Autodesk Inventor part; units mm, degrees
(part 2 of 2)
extrude "Cut10" cut sketch "Sketch17" against normal blind 1.5875 contours A302 L31 | L31 A302 L213 A303 L214 | A300 L31 | L31 A300 L211 A301 L212 | A298 L209 A299 L32 E1 L31 | L31 E1 L32 A299 L210 A298 | L234 A322 L233 L33 | L33 L233 L26 L234 | L26 L233 A323 L234 | L232 A320 L231 L33 | L33 L231 L26 L232 | L26 L231 A321 L232 | L247 A337 L248 L37 | L37 L248 A336 L247 | A332 L243 A333 L43 | L43 A333 L244 A332 | A330 L241 A331 L45 | L45 A331 L242 A330 | A201 L112 A200 L51 | L51 A200 L111 A201 | A181 L92 A180 L51 | L51 A180 L91 A181 | A223 L53 | L53 A223 L134 A222 L133 | A225 L53 | L53 A225 L136 A224 L135 | A162 L73 A163 L74 L54 | L54 A162 | A164 L75 A165 L76 L54 | L54 A164 | A207 L118 A206 L52 | L52 A206 L117 A207 | A187 L98 A186 L52 | L52 A186 L97 A187 | A155 L66 A154 L65 | A173 L84 A172 L83 | A175 L86 A174 L85 | A183 L94 A182 L93 | A185 L96 A184 L95 | A193 L104 A192 L103 | A195 L106 A194 L105 | A203 L114 A202 L113 | A205 L116 A204 L115 | A213 L124 A212 L123 | A215 L126 A214 L125 | A233 L144 A232 L143 | A243 L154 A242 L153 | A245 L156 A244 L155 | A263 L174 A262 L173 | A265 L176 A264 L175 | A283 L194 A282 L193 | A285 L196 A284 L195 | A295 L206 A294 L205 | A309 L220 A308 L219 | A315 L226 A314 L225 | A329 L240 A328 L239 | A335 L246 A334 L245 | A339 L250 A338 L249 | A341 L252 A340 L251 | A343 L254 A342 L253 | A345 L256 A344 L255 | A347 L258 A346 L257 | A349 L260 A348 L259
sketch "Sketch19" plane through (0, 0, 1.5875) normal (0, 0, 1) x (1, 0, 0)
  arc A0 (-129.1273, 301.498) -> (-129.1273, 261.3025) centre (-129.1273, 281.4002) ccw projected
  line L0 (-129.1273, 301.498) -> (-112.1728, 301.498) projected
  arc A1 (-112.1728, 261.3025) -> (-112.1728, 301.498) centre (-112.1728, 281.4002) ccw projected
  line L1 (-112.1728, 261.3025) -> (-129.1273, 261.3025) projected
  arc A2 (-192.6273, 301.498) -> (-192.6273, 261.3025) centre (-192.6273, 281.4002) ccw projected
  line L2 (-192.6273, 301.498) -> (-175.6728, 301.498) projected
  arc A3 (-175.6728, 261.3025) -> (-175.6728, 301.498) centre (-175.6728, 281.4002) ccw projected
  line L3 (-175.6728, 261.3025) -> (-192.6273, 261.3025) projected
  arc A4 (-192.6273, 394.589) -> (-192.6273, 354.3935) centre (-192.6273, 374.4912) ccw projected
  line L4 (-192.6273, 394.589) -> (-175.6728, 394.589) projected
  arc A5 (-175.6728, 354.3935) -> (-175.6728, 394.589) centre (-175.6728, 374.4912) ccw projected
  line L5 (-175.6728, 354.3935) -> (-192.6273, 354.3935) projected
  arc A6 (-65.6273, 208.407) -> (-65.6273, 168.2115) centre (-65.6273, 188.3092) ccw projected
  line L6 (-65.6273, 208.407) -> (-48.6728, 208.407) projected
  arc A7 (-48.6728, 168.2115) -> (-48.6728, 208.407) centre (-48.6727, 188.3092) ccw projected
  line L7 (-48.6728, 168.2115) -> (-65.6273, 168.2115) projected
  arc A8 (-65.6273, 301.498) -> (-65.6273, 261.3025) centre (-65.6273, 281.4002) ccw projected
  line L8 (-65.6273, 301.498) -> (-48.6728, 301.498) projected
  arc A9 (-48.6728, 261.3025) -> (-48.6728, 301.498) centre (-48.6727, 281.4002) ccw projected
  line L9 (-48.6728, 261.3025) -> (-65.6273, 261.3025) projected
  arc A10 (-65.6273, 394.589) -> (-65.6273, 354.3935) centre (-65.6273, 374.4913) ccw projected
  line L10 (-65.6273, 394.589) -> (-48.6728, 394.589) projected
  arc A11 (-48.6728, 354.3935) -> (-48.6728, 394.589) centre (-48.6728, 374.4913) ccw projected
  line L11 (-48.6728, 354.3935) -> (-65.6273, 354.3935) projected
  arc A12 (-65.6273, 487.68) -> (-65.6273, 447.4845) centre (-65.6273, 467.5823) ccw projected
  line L12 (-65.6273, 487.68) -> (-48.6728, 487.68) projected
  arc A13 (-48.6728, 447.4845) -> (-48.6728, 487.68) centre (-48.6728, 467.5823) ccw projected
  line L13 (-48.6728, 447.4845) -> (-65.6273, 447.4845) projected
  arc A14 (-129.1273, 115.316) -> (-129.1273, 75.1205) centre (-129.1273, 95.2182) ccw projected
  line L14 (-129.1273, 115.316) -> (-112.1728, 115.316) projected
  arc A15 (-112.1728, 75.1205) -> (-112.1728, 115.316) centre (-112.1728, 95.2182) ccw projected
  line L15 (-112.1728, 75.1205) -> (-129.1273, 75.1205) projected
  arc A16 (-129.1273, 487.68) -> (-129.1273, 447.4845) centre (-129.1273, 467.5822) ccw projected
  line L16 (-129.1273, 487.68) -> (-112.1728, 487.68) projected
  arc A17 (-112.1728, 447.4845) -> (-112.1728, 487.68) centre (-112.1728, 467.5822) ccw projected
  line L17 (-112.1728, 447.4845) -> (-129.1273, 447.4845) projected
  arc A18 (-192.6273, 487.68) -> (-192.6273, 447.4845) centre (-192.6273, 467.5822) ccw projected
  line L18 (-192.6273, 487.68) -> (-175.6728, 487.68) projected
  arc A19 (-175.6728, 447.4845) -> (-175.6728, 487.68) centre (-175.6728, 467.5822) ccw projected
  line L19 (-175.6728, 447.4845) -> (-192.6273, 447.4845) projected
  arc A20 (-256.1273, 301.498) -> (-256.1273, 261.3025) centre (-256.1273, 281.4002) ccw projected
  line L20 (-256.1273, 301.498) -> (-239.1728, 301.498) projected
  arc A21 (-239.1728, 261.3025) -> (-239.1728, 301.498) centre (-239.1728, 281.4002) ccw projected
  line L21 (-239.1728, 261.3025) -> (-256.1273, 261.3025) projected
  arc A22 (-319.6273, 301.498) -> (-319.6273, 261.3025) centre (-319.6273, 281.4002) ccw projected
  line L22 (-319.6273, 301.498) -> (-302.6728, 301.498) projected
  arc A23 (-302.6728, 261.3025) -> (-302.6728, 301.498) centre (-302.6728, 281.4002) ccw projected
  line L23 (-302.6728, 261.3025) -> (-319.6273, 261.3025) projected
  arc A24 (-383.1273, 301.498) -> (-383.1273, 261.3025) centre (-383.1273, 281.4002) ccw projected
  line L24 (-383.1273, 301.498) -> (-366.1728, 301.498) projected
  arc A25 (-366.1728, 261.3025) -> (-366.1728, 301.498) centre (-366.1728, 281.4002) ccw projected
  line L25 (-366.1728, 261.3025) -> (-383.1273, 261.3025) projected
  arc A26 (-446.6273, 254.9525) -> (-446.6273, 214.757) centre (-446.6273, 234.8547) ccw projected
  line L26 (-446.6273, 254.9525) -> (-429.6728, 254.9525) projected
  arc A27 (-429.6728, 214.757) -> (-429.6728, 254.9525) centre (-429.6728, 234.8547) ccw projected
  line L27 (-429.6728, 214.757) -> (-446.6273, 214.757) projected
  arc A28 (-446.6273, 487.68) -> (-446.6273, 447.4845) centre (-446.6273, 467.5822) ccw projected
  line L28 (-446.6273, 487.68) -> (-429.6728, 487.68) projected
  arc A29 (-429.6728, 447.4845) -> (-429.6728, 487.68) centre (-429.6728, 467.5822) ccw projected
  line L29 (-429.6728, 447.4845) -> (-446.6273, 447.4845) projected
  arc A30 (-510.1273, 208.407) -> (-510.1273, 168.2115) centre (-510.1273, 188.3092) ccw projected
  line L30 (-510.1273, 208.407) -> (-493.1728, 208.407) projected
  arc A31 (-493.1728, 168.2115) -> (-493.1728, 208.407) centre (-493.1727, 188.3092) ccw projected
  line L31 (-493.1728, 168.2115) -> (-510.1273, 168.2115) projected
  arc A32 (-510.1273, 301.498) -> (-510.1273, 261.3025) centre (-510.1273, 281.4002) ccw projected
  line L32 (-510.1273, 301.498) -> (-493.1728, 301.498) projected
  arc A33 (-493.1728, 261.3025) -> (-493.1728, 301.498) centre (-493.1728, 281.4002) ccw projected
  line L33 (-493.1728, 261.3025) -> (-510.1273, 261.3025) projected
  arc A34 (-510.1273, 487.68) -> (-510.1273, 447.4845) centre (-510.1273, 467.5822) ccw projected
  line L34 (-510.1273, 487.68) -> (-493.1728, 487.68) projected
  arc A35 (-493.1728, 447.4845) -> (-493.1728, 487.68) centre (-493.1728, 467.5822) ccw projected
  line L35 (-493.1728, 447.4845) -> (-510.1273, 447.4845) projected
  arc A36 (-573.6273, 208.407) -> (-573.6273, 168.2115) centre (-573.6273, 188.3092) ccw projected
  line L36 (-573.6273, 208.407) -> (-556.6728, 208.407) projected
  arc A37 (-556.6728, 168.2115) -> (-556.6728, 208.407) centre (-556.6727, 188.3092) ccw projected
  line L37 (-556.6728, 168.2115) -> (-573.6273, 168.2115) projected
  arc A38 (-573.6273, 301.498) -> (-573.6273, 261.3025) centre (-573.6273, 281.4002) ccw projected
  line L38 (-573.6273, 301.498) -> (-556.6728, 301.498) projected
  arc A39 (-556.6728, 261.3025) -> (-556.6728, 301.498) centre (-556.6728, 281.4002) ccw projected
  line L39 (-556.6728, 261.3025) -> (-573.6273, 261.3025) projected
  arc A40 (-573.6273, 487.68) -> (-573.6273, 447.4845) centre (-573.6273, 467.5822) ccw projected
  line L40 (-573.6273, 487.68) -> (-556.6728, 487.68) projected
  arc A41 (-556.6728, 447.4845) -> (-556.6728, 487.68) centre (-556.6728, 467.5822) ccw projected
  line L41 (-556.6728, 447.4845) -> (-573.6273, 447.4845) projected
  arc A42 (-637.1273, 254.9525) -> (-637.1273, 214.757) centre (-637.1273, 234.8547) ccw projected
  line L42 (-637.1273, 254.9525) -> (-620.1728, 254.9525) projected
  arc A43 (-620.1728, 214.757) -> (-620.1728, 254.9525) centre (-620.1727, 234.8547) ccw projected
  line L43 (-620.1728, 214.757) -> (-637.1273, 214.757) projected
  arc A44 (-637.1273, 487.68) -> (-637.1273, 447.4845) centre (-637.1273, 467.5822) ccw projected
  line L44 (-637.1273, 487.68) -> (-620.1728, 487.68) projected
  arc A45 (-620.1728, 447.4845) -> (-620.1728, 487.68) centre (-620.1728, 467.5822) ccw projected
  line L45 (-620.1728, 447.4845) -> (-637.1273, 447.4845) projected
  arc A46 (-637.1273, 301.498) -> (-637.1273, 261.3025) centre (-637.1273, 281.4002) ccw projected
  line L46 (-637.1273, 301.498) -> (-620.1728, 301.498) projected
  arc A47 (-620.1728, 261.3025) -> (-620.1728, 301.498) centre (-620.1727, 281.4002) ccw projected
  line L47 (-620.1728, 261.3025) -> (-637.1273, 261.3025) projected
  arc A48 (-637.1272, 68.7705) -> (-637.1272, 28.575) centre (-637.1272, 48.6727) ccw projected
  line L48 (-637.1272, 68.7705) -> (-620.1728, 68.7705) projected
  arc A49 (-620.1728, 28.575) -> (-620.1728, 68.7705) centre (-620.1727, 48.6727) ccw projected
  line L49 (-620.1728, 28.575) -> (-637.1272, 28.575) projected
  arc A50 (-573.6273, 348.0435) -> (-573.6273, 307.848) centre (-573.6273, 327.9457) ccw projected
  line L50 (-573.6273, 348.0435) -> (-556.6728, 348.0435) projected
  arc A51 (-556.6728, 307.848) -> (-556.6728, 348.0435) centre (-556.6728, 327.9457) ccw projected
  line L51 (-556.6728, 307.848) -> (-573.6273, 307.848) projected
  arc A52 (-573.6273, 254.9525) -> (-573.6273, 214.757) centre (-573.6273, 234.8547) ccw projected
  line L52 (-573.6273, 254.9525) -> (-556.6728, 254.9525) projected
  arc A53 (-556.6728, 214.757) -> (-556.6728, 254.9525) centre (-556.6727, 234.8547) ccw projected
  line L53 (-556.6728, 214.757) -> (-573.6273, 214.757) projected
  arc A54 (-573.6273, 68.7705) -> (-573.6273, 28.575) centre (-573.6273, 48.6727) ccw projected
  line L54 (-573.6273, 68.7705) -> (-556.6728, 68.7705) projected
  arc A55 (-556.6728, 28.575) -> (-556.6728, 68.7705) centre (-556.6727, 48.6727) ccw projected
  line L55 (-556.6728, 28.575) -> (-573.6273, 28.575) projected
  arc A56 (-510.1273, 348.0435) -> (-510.1273, 307.848) centre (-510.1273, 327.9457) ccw projected
  line L56 (-510.1273, 348.0435) -> (-493.1728, 348.0435) projected
  arc A57 (-493.1728, 307.848) -> (-493.1728, 348.0435) centre (-493.1728, 327.9457) ccw projected
  line L57 (-493.1728, 307.848) -> (-510.1273, 307.848) projected
  arc A58 (-510.1273, 254.9525) -> (-510.1273, 214.757) centre (-510.1273, 234.8547) ccw projected
  line L58 (-510.1273, 254.9525) -> (-493.1728, 254.9525) projected
  arc A59 (-493.1728, 214.757) -> (-493.1728, 254.9525) centre (-493.1727, 234.8547) ccw projected
  line L59 (-493.1728, 214.757) -> (-510.1273, 214.757) projected
  arc A60 (-510.1272, 68.7705) -> (-510.1272, 28.575) centre (-510.1272, 48.6727) ccw projected
  line L60 (-510.1272, 68.7705) -> (-493.1728, 68.7705) projected
  arc A61 (-493.1728, 28.575) -> (-493.1728, 68.7705) centre (-493.1727, 48.6727) ccw projected
  line L61 (-493.1728, 28.575) -> (-510.1272, 28.575) projected
  arc A62 (-446.6273, 301.498) -> (-446.6273, 261.3025) centre (-446.6273, 281.4002) ccw projected
  line L62 (-446.6273, 301.498) -> (-429.6728, 301.498) projected
  arc A63 (-429.6728, 261.3025) -> (-429.6728, 301.498) centre (-429.6728, 281.4002) ccw projected
  line L63 (-429.6728, 261.3025) -> (-446.6273, 261.3025) projected
  arc A64 (-446.6272, 68.7705) -> (-446.6272, 28.575) centre (-446.6272, 48.6727) ccw projected
  line L64 (-446.6272, 68.7705) -> (-429.6728, 68.7705) projected
  arc A65 (-429.6728, 28.575) -> (-429.6728, 68.7705) centre (-429.6728, 48.6727) ccw projected
  line L65 (-429.6728, 28.575) -> (-446.6272, 28.575) projected
  arc A66 (-383.1273, 254.9525) -> (-383.1273, 214.757) centre (-383.1273, 234.8547) ccw projected
  line L66 (-383.1273, 254.9525) -> (-366.1728, 254.9525) projected
  arc A67 (-366.1728, 214.757) -> (-366.1728, 254.9525) centre (-366.1728, 234.8547) ccw projected
  line L67 (-366.1728, 214.757) -> (-383.1273, 214.757) projected
  arc A68 (-319.6273, 254.9525) -> (-319.6273, 214.757) centre (-319.6273, 234.8547) ccw projected
  line L68 (-319.6273, 254.9525) -> (-302.6728, 254.9525) projected
  arc A69 (-302.6728, 214.757) -> (-302.6728, 254.9525) centre (-302.6727, 234.8547) ccw projected
  line L69 (-302.6728, 214.757) -> (-319.6273, 214.757) projected
  arc A70 (-256.1273, 254.9525) -> (-256.1273, 214.757) centre (-256.1273, 234.8547) ccw projected
  line L70 (-256.1273, 254.9525) -> (-239.1728, 254.9525) projected
  arc A71 (-239.1728, 214.757) -> (-239.1728, 254.9525) centre (-239.1728, 234.8547) ccw projected
  line L71 (-239.1728, 214.757) -> (-256.1273, 214.757) projected
  arc A72 (-192.6273, 161.8615) -> (-192.6273, 121.666) centre (-192.6273, 141.7637) ccw projected
  line L72 (-192.6273, 161.8615) -> (-175.6728, 161.8615) projected
  arc A73 (-175.6728, 121.666) -> (-175.6728, 161.8615) centre (-175.6728, 141.7637) ccw projected
  line L73 (-175.6728, 121.666) -> (-192.6273, 121.666) projected
  arc A74 (-129.1273, 161.8615) -> (-129.1273, 121.666) centre (-129.1273, 141.7637) ccw projected
  line L74 (-129.1273, 161.8615) -> (-112.1728, 161.8615) projected
  arc A75 (-112.1728, 121.666) -> (-112.1728, 161.8615) centre (-112.1728, 141.7637) ccw projected
  line L75 (-112.1728, 121.666) -> (-129.1273, 121.666) projected
  arc A76 (-129.1272, 68.7705) -> (-129.1272, 28.575) centre (-129.1272, 48.6727) ccw projected
  line L76 (-129.1272, 68.7705) -> (-112.1728, 68.7705) projected
  arc A77 (-112.1728, 28.575) -> (-112.1728, 68.7705) centre (-112.1727, 48.6727) ccw projected
  line L77 (-112.1728, 28.575) -> (-129.1272, 28.575) projected
  arc A78 (-65.6273, 441.1345) -> (-65.6273, 400.939) centre (-65.6273, 421.0368) ccw projected
  line L78 (-65.6273, 441.1345) -> (-48.6728, 441.1345) projected
  arc A79 (-48.6728, 400.939) -> (-48.6728, 441.1345) centre (-48.6728, 421.0368) ccw projected
  line L79 (-48.6728, 400.939) -> (-65.6273, 400.939) projected
  arc A80 (-65.6273, 348.0435) -> (-65.6273, 307.848) centre (-65.6273, 327.9458) ccw projected
  line L80 (-65.6273, 348.0435) -> (-48.6728, 348.0435) projected
  arc A81 (-48.6728, 307.848) -> (-48.6728, 348.0435) centre (-48.6727, 327.9458) ccw projected
  line L81 (-48.6728, 307.848) -> (-65.6273, 307.848) projected
  arc A82 (-65.6273, 254.9525) -> (-65.6273, 214.757) centre (-65.6273, 234.8547) ccw projected
  line L82 (-65.6273, 254.9525) -> (-48.6728, 254.9525) projected
  arc A83 (-48.6728, 214.757) -> (-48.6728, 254.9525) centre (-48.6727, 234.8547) ccw projected
  line L83 (-48.6728, 214.757) -> (-65.6273, 214.757) projected
  arc A84 (-65.6273, 161.8615) -> (-65.6273, 121.666) centre (-65.6273, 141.7638) ccw projected
  line L84 (-65.6273, 161.8615) -> (-48.6728, 161.8615) projected
  arc A85 (-48.6728, 121.666) -> (-48.6728, 161.8615) centre (-48.6727, 141.7638) ccw projected
  line L85 (-48.6728, 121.666) -> (-65.6273, 121.666) projected
  arc A86 (-192.6273, 348.0435) -> (-192.6273, 307.848) centre (-192.6273, 327.9457) ccw projected
  line L86 (-192.6273, 348.0435) -> (-175.6728, 348.0435) projected
  arc A87 (-175.6728, 307.848) -> (-175.6728, 348.0435) centre (-175.6728, 327.9457) ccw projected
  line L87 (-175.6728, 307.848) -> (-192.6273, 307.848) projected
  arc A88 (-129.1273, 348.0435) -> (-129.1273, 307.848) centre (-129.1273, 327.9457) ccw projected
  line L88 (-129.1273, 348.0435) -> (-112.1728, 348.0435) projected
  arc A89 (-112.1728, 307.848) -> (-112.1728, 348.0435) centre (-112.1728, 327.9457) ccw projected
  line L89 (-112.1728, 307.848) -> (-129.1273, 307.848) projected
  circle A90 centre (-435.0722, 321.6304) radius 3.2639 projected
  circle A91 centre (-198.3647, 418.811) radius 2.5119 projected
  circle A92 centre (-446.7241, 420.236) radius 2.1989 projected
  circle A93 centre (-542.5208, 420.236) radius 2.1989 projected
  circle A94 centre (-644.6428, 420.236) radius 2.1989 projected
  circle A95 centre (-593.5881, 357.8965) radius 2.1989 projected
  circle A96 centre (-404.9157, 358.1076) radius 2.1723 projected
  arc A97 (-499.3886, 356.3852) -> (-499.1548, 359.6218) centre (-497.7914, 357.8965) ccw projected
  arc A98 (-499.1548, 359.6218) -> (-499.3886, 356.3852) centre (-500.7124, 358.1076) ccw projected
  circle A99 centre (-602.8344, 358.1076) radius 2.1723 projected
  circle A100 centre (-455.983, 420.0249) radius 2.1723 projected
  circle A101 centre (-551.7797, 420.0249) radius 2.1723 projected
  circle A102 centre (-131.6773, 209.9079) radius 3.5177 projected
  circle A103 centre (-644.6222, 194.6304) radius 3.2639 projected
  circle A104 centre (-57.15, 98.044) radius 2.4116 projected
  circle A105 centre (-197.0948, 59.563) radius 2.4116 projected
  circle A106 centre (-196.794, 254.6594) radius 2.2655 projected
  circle A107 centre (-542.5208, 158.3585) radius 2.1989 projected
  circle A108 centre (-446.7241, 96.019) radius 2.1989 projected
  circle A109 centre (-542.5208, 96.019) radius 2.1989 projected
  circle A110 centre (-644.6428, 96.019) radius 2.1989 projected
  circle A111 centre (-455.983, 96.2301) radius 2.1723 projected
  arc A112 (-499.3886, 94.5077) -> (-499.1548, 97.7443) centre (-497.7914, 96.019) ccw projected
  arc A113 (-499.1548, 97.7443) -> (-499.3886, 94.5077) centre (-500.7124, 96.2301) ccw projected
  circle A114 centre (-404.9157, 158.1474) radius 2.1723 projected
  arc A115 (-499.1548, 156.6332) -> (-499.3886, 159.8698) centre (-497.7914, 158.3585) ccw projected
  arc A116 (-499.3886, 159.8698) -> (-499.1548, 156.6332) centre (-500.7124, 158.1474) ccw projected
  circle A117 centre (-602.8344, 158.1474) radius 2.1723 projected
  circle A118 centre (-551.7797, 158.1474) radius 2.1723 projected
  circle A119 centre (-455.983, 158.1474) radius 2.1723 projected
  circle A120 centre (-404.9157, 96.2301) radius 2.1723 projected
  circle A121 centre (-551.7797, 96.2301) radius 2.1723 projected
  circle A122 centre (-602.8344, 96.2301) radius 2.1723 projected
  circle A123 centre (-593.5881, 96.019) radius 2.1989 projected
  circle A124 centre (-593.5881, 158.3585) radius 2.1989 projected
  circle A125 centre (-446.7241, 158.3585) radius 2.1989 projected
  circle A126 centre (-644.6428, 158.3585) radius 2.1989 projected
  circle A127 centre (-197.0948, 95.631) radius 2.4116 projected
  circle A128 centre (-57.15, 57.15) radius 2.4116 projected
  circle A129 centre (-435.0722, 194.6304) radius 3.2639 projected
  circle A130 centre (-187.6385, 209.9079) radius 3.5177 projected
  circle A131 centre (-602.8344, 420.0249) radius 2.1723 projected
  arc A132 (-499.1548, 418.5107) -> (-499.3886, 421.7473) centre (-497.7914, 420.236) ccw projected
  arc A133 (-499.3886, 421.7473) -> (-499.1548, 418.5107) centre (-500.7124, 420.0249) ccw projected
  circle A134 centre (-404.9157, 420.0249) radius 2.1723 projected
  circle A135 centre (-551.7797, 358.1076) radius 2.1723 projected
  circle A136 centre (-455.983, 358.1076) radius 2.1723 projected
  circle A137 centre (-644.6428, 357.8965) radius 2.1989 projected
  circle A138 centre (-542.5208, 357.8965) radius 2.1989 projected
  circle A139 centre (-446.7241, 357.8965) radius 2.1989 projected
  circle A140 centre (-593.5881, 420.236) radius 2.1989 projected
  circle A141 centre (-133.294, 368.9594) radius 2.2479 projected
  circle A142 centre (-151.1207, 418.811) radius 2.5119 projected
  circle A143 centre (-644.6222, 321.6304) radius 3.2639 projected
  circle A144 centre (-12.7, 486.7275) radius 2.0701 projected
  circle A145 centre (-12.7, 461.3275) radius 2.0701 projected
  circle A146 centre (-12.7, 435.9275) radius 2.0701 projected
  circle A147 centre (-12.7, 410.5275) radius 2.0701 projected
  circle A148 centre (-12.7, 385.1275) radius 2.0701 projected
  circle A149 centre (-12.7, 359.7275) radius 2.0701 projected
  circle A150 centre (-12.7, 334.3275) radius 2.0701 projected
  circle A151 centre (-12.7, 308.9275) radius 2.0701 projected
  circle A152 centre (-12.7, 283.5275) radius 2.0701 projected
  circle A153 centre (-12.7, 258.1275) radius 2.0701 projected
  circle A154 centre (-12.7, 232.7275) radius 2.0701 projected
  circle A155 centre (-12.7, 207.3275) radius 2.0701 projected
  circle A156 centre (-12.7, 181.9275) radius 2.0701 projected
  circle A157 centre (-12.7, 156.5275) radius 2.0701 projected
  circle A158 centre (-12.7, 131.1275) radius 2.0701 projected
  circle A159 centre (-12.7, 105.7275) radius 2.0701 projected
  circle A160 centre (-12.7, 80.3275) radius 2.0701 projected
  circle A161 centre (-12.7, 54.9275) radius 2.0701 projected
  circle A162 centre (-12.7, 29.5275) radius 2.0701 projected
  circle A163 centre (-673.1, 486.7275) radius 2.0701 projected
  circle A164 centre (-673.1, 461.3275) radius 2.0701 projected
  circle A165 centre (-673.1, 435.9275) radius 2.0701 projected
  circle A166 centre (-673.1, 410.5275) radius 2.0701 projected
  circle A167 centre (-673.1, 385.1275) radius 2.0701 projected
  circle A168 centre (-673.1, 359.7275) radius 2.0701 projected
  circle A169 centre (-673.1, 334.3275) radius 2.0701 projected
  circle A170 centre (-673.1, 308.9275) radius 2.0701 projected
  circle A171 centre (-673.1, 283.5275) radius 2.0701 projected
  circle A172 centre (-673.1, 258.1275) radius 2.0701 projected
  circle A173 centre (-673.1, 232.7275) radius 2.0701 projected
  circle A174 centre (-673.1, 207.3275) radius 2.0701 projected
  circle A175 centre (-673.1, 181.9275) radius 2.0701 projected
  circle A176 centre (-673.1, 156.5275) radius 2.0701 projected
  circle A177 centre (-673.1, 131.1275) radius 2.0701 projected
  circle A178 centre (-673.1, 105.7275) radius 2.0701 projected
  circle A179 centre (-673.1, 80.3275) radius 2.0701 projected
  circle A180 centre (-673.1, 54.9275) radius 2.0701 projected
  circle A181 centre (-673.1, 29.5275) radius 2.0701 projected
  line L90 (-252.73, 490.855) -> (-252.73, 332.105) projected
  line L91 (-252.73, 332.105) -> (-392.43, 332.105) projected
  line L92 (-392.43, 332.105) -> (-392.43, 490.855) projected
  line L93 (-392.43, 490.855) -> (-252.73, 490.855) projected
  line L94 (-252.73, 25.4) -> (-392.43, 25.4) projected
  line L95 (-392.43, 25.4) -> (-392.43, 184.15) projected
  line L96 (-392.43, 184.15) -> (-252.73, 184.15) projected
  line L97 (-252.73, 184.15) -> (-252.73, 25.4) projected
  circle A182 centre (-12.7, 503.555) radius 2.0828 projected
  circle A183 centre (-12.7, 12.7) radius 2.0828 projected
  circle A184 centre (-38.1, 503.555) radius 2.0828 projected
  circle A185 centre (-38.1, 12.7) radius 2.0828 projected
  circle A186 centre (-63.5, 503.555) radius 2.0828 projected
  circle A187 centre (-63.5, 12.7) radius 2.0828 projected
  circle A188 centre (-88.9, 503.555) radius 2.0828 projected
  circle A189 centre (-88.9, 12.7) radius 2.0828 projected
  circle A190 centre (-114.3, 503.555) radius 2.0828 projected
  circle A191 centre (-114.3, 12.7) radius 2.0828 projected
  circle A192 centre (-139.7, 503.555) radius 2.0828 projected
  circle A193 centre (-139.7, 12.7) radius 2.0828 projected
  circle A194 centre (-165.1, 503.555) radius 2.0828 projected
  circle A195 centre (-165.1, 12.7) radius 2.0828 projected
  circle A196 centre (-190.5, 503.555) radius 2.0828 projected
  circle A197 centre (-190.5, 12.7) radius 2.0828 projected
  circle A198 centre (-215.9, 503.555) radius 2.0828 projected
  circle A199 centre (-215.9, 12.7) radius 2.0828 projected
  circle A200 centre (-241.3, 503.555) radius 2.0828 projected
  circle A201 centre (-241.3, 12.7) radius 2.0828 projected
  circle A202 centre (-266.7, 503.555) radius 2.0828 projected
  circle A203 centre (-266.7, 12.7) radius 2.0828 projected
  circle A204 centre (-292.1, 503.555) radius 2.0828 projected
  circle A205 centre (-292.1, 12.7) radius 2.0828 projected
  circle A206 centre (-317.5, 503.555) radius 2.0828 projected
  circle A207 centre (-317.5, 12.7) radius 2.0828 projected
  circle A208 centre (-342.9, 503.555) radius 2.0828 projected
  circle A209 centre (-342.9, 12.7) radius 2.0828 projected
  circle A210 centre (-368.3, 503.555) radius 2.0828 projected
  circle A211 centre (-368.3, 12.7) radius 2.0828 projected
  circle A212 centre (-393.7, 503.555) radius 2.0828 projected
  circle A213 centre (-393.7, 12.7) radius 2.0828 projected
  circle A214 centre (-419.1, 503.555) radius 2.0828 projected
  circle A215 centre (-419.1, 12.7) radius 2.0828 projected
  circle A216 centre (-444.5, 503.555) radius 2.0828 projected
  circle A217 centre (-444.5, 12.7) radius 2.0828 projected
  circle A218 centre (-469.9, 503.555) radius 2.0828 projected
  circle A219 centre (-469.9, 12.7) radius 2.0828 projected
  circle A220 centre (-495.3, 503.555) radius 2.0828 projected
  circle A221 centre (-495.3, 12.7) radius 2.0828 projected
  circle A222 centre (-520.7, 503.555) radius 2.0828 projected
  circle A223 centre (-520.7, 12.7) radius 2.0828 projected
  circle A224 centre (-546.1, 503.555) radius 2.0828 projected
  circle A225 centre (-546.1, 12.7) radius 2.0828 projected
  circle A226 centre (-571.5, 503.555) radius 2.0828 projected
  circle A227 centre (-571.5, 12.7) radius 2.0828 projected
  circle A228 centre (-596.9, 503.555) radius 2.0828 projected
  circle A229 centre (-596.9, 12.7) radius 2.0828 projected
  circle A230 centre (-622.3, 503.555) radius 2.0828 projected
  circle A231 centre (-622.3, 12.7) radius 2.0828 projected
  circle A232 centre (-647.7, 503.555) radius 2.0828 projected
  circle A233 centre (-647.7, 12.7) radius 2.0828 projected
  circle A234 centre (-673.1, 503.555) radius 2.0828 projected
  circle A235 centre (-673.1, 12.7) radius 2.0828 projected
  line L98 (-685.8, 0) -> (-685.8, 516.255) projected
  line L99 (0, 0) -> (-685.8, 0) projected
  line L100 (0, 516.255) -> (0, 0) projected
  line L101 (-685.8, 516.255) -> (0, 516.255) projected
equation "\"d17\" = Thickness"
equation "\"d65\" = Thickness"
equation "\"BendRadius\" = Thickness"
equation "\"BendReliefWidth\" = Thickness"
equation "\"BendReliefDepth\" = 0.5 * Thickness"
equation "\"CornerReliefSize\" = 4 * Thickness"
equation "\"MinimumRemnant\" = 2 * Thickness"
equation "\"TransitionRadius\" = BendRadius"
equation "\"JacobiRadiusSize\" = Thickness"
equation "\"GapSize\" = Thickness"
equation "\"d2\" = BendRadius"
equation "\"Thickness\" = 1.5875"
body "Solid1"
